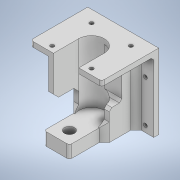
# Autodesk Inventor part: suporte barra motor 2
Saved by Autodesk Inventor 2022 (Build 260153000, 153)
## iProperties
Created: 2022-02-16
Part Number: suporte barra motor 2
Material: Genérico
Document SubType Name: Modeling
Designer: mathe
Density: 1 g/cm^3
Appearance: Padrão
Author: mathe
Autodesk Inventor part; units mm, degrees
ref_plane "YZ Plane" through (0, 0, 0) normal (1, 0, 0) x (0, 1, 0)
ref_plane "XZ Plane" through (0, 0, 0) normal (0, 1, 0) x (-1, 0, 0)
ref_plane "XY Plane" through (0, 0, 0) normal (0, 0, 1) x (1, 0, 0)
sketch "Esboço1" plane through (0, 0, 0) normal (0, 0, 1) x (1, 0, 0)
  line L0 (0, 0) -> (56, 0)
  line L1 (56, 0) -> (56, 10)
  line L2 (56, 10) -> (0, 10)
  line L3 (0, 10) -> (0, 0)
  line L4 (18, 10) -> (38, 10)
  line L5 (38, 10) -> (38, 0)
  line L6 (38, 0) -> (18, 0)
  line L7 (18, 0) -> (18, 10)
  line L8 (18, 10) -> (38, 0) construction
  line L9 (38, 10) -> (18, 0) construction
  point P0 (28, 5)
  dimension "d0" = 56
  dimension "d1" = 10
  dimension "d2" = 20
  constraints: 20 end point, 4 parallel, 2 horizontal, 2 midpoint, 2 perpendicular, 1 point on line
  measures "d0" distance of L2.end L1.end
  measures "d1" distance of L1.end L0.end
  measures "d2" distance of L5.end L6.end
extrude "Extrusão1" add sketch "Esboço1" along normal blind 4 contours L3 L2 L7 L0 | L5 L2 L1 L0
extrude "Extrusão2" add sketch "Esboço1" along normal blind 52.426 contours L7 L2 L5 L0
sketch "Esboço2" plane through (0, 10, 0) normal (0, 1, 0) x (1, 0, 0)
  line L0 (38, -52.426) -> (18, -52.426) projected
  point P0 (0, 0)
  point P1 (28, -42.426)
  point P2 (33, -52.426)
  point P3 (23, -52.426)
  dimension "d24" = 10
  measures "d24" distance from line of L0 point (28, -42.426)
hole "Furo1" at (28, 10, 42.426) direction (0, -1, 0) diameter 8 end through all
sketch "Esboço3" plane through (0, 0, 4) normal (0, 0, 1) x (1, 0, 0)
  point P0 (0, 0)
  point P1 (6.5, 5)
  point P2 (49.5, 5)
hole "Furo2" at (6.5, 5, 4) at (49.5, 5, 4) direction (0, 0, -1) diameter 3 end through all
sketch "Esboço4" plane through (0, 10, 0) normal (0, 1, 0) x (1, 0, 0)
  line L0 (56, 0) -> (0, 0) projected
  line L1 (0, 0) -> (56, 0)
  line L2 (56, 0) -> (56, -25)
  line L3 (56, -25) -> (0, -25)
  line L4 (0, -25) -> (0, 0)
  dimension "d25" = 25
  constraints: 8 end point, 2 parallel, 1 horizontal, 1 perpendicular
  measures "d25" distance of L1.end L2.end
extrude "Extrusão3" add sketch "Esboço4" along normal blind 39
sketch "Esboço5" plane through (0, 49, 0) normal (0, 1, 0) x (1, 0, 0)
  line L0 (0, -25) -> (56, -25) projected
  circle A0 centre (28, -25) radius 10
  line L1 (38, -4) -> (38, -52.426) projected
  point P0 (0, 0)
  point P1 (38, -9)
  point P2 (38, -47.426)
  point P3 (38, -25)
  point P4 (18, -25)
  constraints: 1 centre point, 1 midpoint, 1 tangent
extrude "Extrusão4" cut sketch "Esboço5" against normal blind 22 contours A0 L0 picked at (30.9515, -23.4509)
sketch "Esboço6" plane through (0, 49, 0) normal (0, 1, 0) x (1, 0, 0)
  arc A0 (38, -25) -> (18, -25) centre (28, -25) ccw projected
  line L0 (18, -25) -> (18, -52.426) projected
  line L1 (0, -25) -> (18, -25)
  line L2 (18, -25) -> (18, -45)
  line L3 (18, -45) -> (0, -45)
  line L4 (0, -45) -> (0, -25)
  line L5 (38, -25) -> (38, -52.426) projected
  line L6 (56, -25) -> (38, -25)
  line L7 (38, -25) -> (38, -45)
  line L8 (38, -45) -> (56, -45)
  line L9 (56, -45) -> (56, -25)
  circle A1 centre (43.5, -9.5) radius 1.5
  circle A2 centre (12.5, -9.5) radius 1.5
  circle A3 centre (12.5, -40.5) radius 1.5
  circle A4 centre (43.5, -40.5) radius 1.5
  point P0 (0, 0)
  point P1 (18, -47.426)
  point P2 (38, -47.426)
  dimension "d30" = 15.5
  dimension "d31" = 15.5
  dimension "d32" = 15.5
  dimension "d33" = 15.5
  dimension "d34" = 20
  dimension "d37" = 3
  dimension "d38" = 3
  dimension "d39" = 3
  dimension "d40" = 3
  dimension "d103" = 15.5
  dimension "d104" = 15.5
  constraints: 16 end point, 4 centre point, 4 coincident, 4 parallel, 3 point on line, 2 horizontal, 2 perpendicular
  measures "d30" horizontal distance of point (43.5, -9.5) A0.centre
  measures "d31" horizontal distance of A0.centre point (43.5, -9.5)
  measures "d32" horizontal distance of point (12.5, -9.5) A0.centre
  measures "d33" horizontal distance of A0.centre point (12.5, -9.5)
  measures "d34" distance of L1.end L2.end
  measures "d37" diameter of A1
  measures "d38" diameter of A2
  measures "d39" diameter of A3
  measures "d40" diameter of A4
  measures "d103" distance from line of L1 A3.centre
  measures "d104" distance from line of L6 A4.centre
extrude "Extrusão5" add sketch "Esboço6" against normal up to surface (22 mm away) contours L0 L3 L4 L1 | L6 L9 L8 L5 | A3 | A4
extrude "Extrusão6" cut sketch "Esboço6" against normal blind 20 contours A1 | A2 | A3 | A4
sketch "Esboço7" plane through (0, 0, 0) normal (-1, 0, 0) x (0, 0, 1)
  line L0 (4, 0) -> (4, 10) projected
  line L1 (45, 49) -> (45, 27) projected
  line L2 (4, 10) -> (45, 10)
  line L3 (45, 10) -> (45, 45)
  line L4 (45, 45) -> (4, 45)
  line L5 (4, 45) -> (4, 10)
  line L6 (0, 49) -> (45, 49) projected
  point P0 (0, 0)
  dimension "d43" = 4
  constraints: 8 end point, 2 parallel, 1 horizontal, 1 perpendicular, 1 point on line
  measures "d43" distance between parallel lines of L6 L4
extrude "Extrusão7" cut sketch "Esboço7" against normal blind 14
sketch "Esboço8" plane through (56, 0, 4) normal (1, 0, 0) x (0, 0, -1)
  line L0 (4, 0) -> (0, 0) projected
  line L1 (-41, 49) -> (-41, 27) projected
  line L2 (0, 0) -> (-41, 0)
  line L3 (-41, 0) -> (-41, 45)
  line L4 (-41, 45) -> (0, 45)
  line L5 (0, 45) -> (0, 0)
  line L6 (-41, 49) -> (4, 49) projected
  dimension "d46" = 4
  constraints: 8 end point, 2 parallel, 1 horizontal, 1 perpendicular, 1 point on line
  measures "d46" distance between parallel lines of L6 L4
extrude "Extrusão8" cut sketch "Esboço8" against normal blind 14
sketch "Esboço9" plane through (0, 27, 0) normal (0, 1, 0) x (1, 0, 0)
  line L0 (38, -25) -> (18, -25) projected
  circle A0 centre (28, -25) radius 10
  point P0 (0, 0)
  constraints: 1 centre point, 1 midpoint
extrude "Extrusão9" cut sketch "Esboço9" against normal up to surface (17 mm away) contours L0 A0 picked at (30.9515, -23.4509)
sketch "Esboço10" plane through (0, 10, 0) normal (0, -1, 0) x (1, 0, 0)
  line L0 (18, 25) -> (14, 25) projected
  line L1 (14, 4) -> (14, 9.5) projected
  line L2 (18, 25) -> (14, 25)
  line L3 (14, 25) -> (14, 4)
  line L4 (14, 4) -> (18, 4)
  line L5 (18, 4) -> (18, 25)
  line L6 (38, 25) -> (42, 25) projected
  line L7 (38, 4) -> (56, 4) projected
  line L8 (42, 25) -> (38, 25)
  line L9 (38, 25) -> (38, 4)
  line L10 (38, 4) -> (42, 4)
  line L11 (42, 4) -> (42, 25)
  point P0 (0, 0)
  constraints: 16 end point, 4 parallel, 2 horizontal, 2 perpendicular
extrude "Extrusão10" add sketch "Esboço10" along normal blind 10
chamfer "Chanfro2" distance 4 angle 45 8 edges at (42, 22.5, 4) (38, 5, 25) (18, 5, 25) (14, 22.5, 4) (16, 27, 25) (40, 27, 25) (40, 27, 45) (16, 27, 45)
fillet "Arredondamento1" radius 2 4 edges at (18, 5, 52.426) (38, 5, 52.426) (0, 47, 45) (56, 47, 45)
sketch "Esboço11" plane through (0, 0, 4) normal (0, 0, 1) x (1, 0, 0)
  circle A0 centre (6.5, 5) radius 1.5 projected
  line L0 (6.5, 5) -> (6.5, 38)
  point P0 (0, 0)
  point P1 (49.5, 38)
  dimension "d57" = 33
  constraints: 2 end point, 1 coincident, 1 vertical
  measures "d57" distance of L0.start L0.end
hole "Furo3" at (6.5, 38, 4) at (49.5, 38, 4) direction (0, 0, -1) diameter 3 end through all
sketch "Esboço12" plane through (0, 49, 0) normal (0, 1, 0) x (1, 0, 0)
  line L0 (0, 0) -> (56, 0)
  line L1 (56, 0) -> (56, -45)
  line L2 (56, -45) -> (0, -45)
  line L3 (0, -45) -> (0, 0)
  constraints: 8 end point, 2 parallel, 1 horizontal, 1 perpendicular
extrude "Extrusão11" add sketch "Esboço12" along normal blind 10
fillet "Arredondamento2" radius 2 2 edges at (56, 54, 45) (0, 54, 45)
sketch "Esboço13" plane through (12.5, 45, 9.5) normal (0, -1, 0) x (1, 0, 0)
  circle A0 centre (0, 0) radius 1.5 projected
  circle A1 centre (0, 0) radius 1.5
  circle A2 centre (0, 31) radius 1.5 projected
  circle A3 centre (0, 31) radius 1.5
  circle A4 centre (31, 31) radius 1.5 projected
  circle A5 centre (31, 31) radius 1.5
  circle A6 centre (31, 0) radius 1.5 projected
  circle A7 centre (31, 0) radius 1.5
  point P0 (-12.5, -9.5)
  point P1 (1.5, 0)
  point P2 (1.5, 31)
  point P3 (29.5, 0)
  constraints: 4 coincident, 4 horizontal alignment, 3 centre point, 2 other
extrude "Extrusão12" cut sketch "Esboço13" against normal through all
sketch "Esboço14" plane through (56, 0, 4) normal (1, 0, 0) x (0, 0, -1)
  line L0 (0, 0) -> (0, 45) projected
  line L1 (0, 45) -> (-45.5354, 45)
  line L2 (-45.5354, 45) -> (-45.5354, 55)
  line L3 (-45.5354, 55) -> (0, 55)
  line L4 (0, 55) -> (0, 45)
  line L5 (-39, 59) -> (4, 59) projected
  point P0 (4, 0)
  dimension "d70" = 4
  constraints: 8 end point, 2 parallel, 1 horizontal, 1 perpendicular
  measures "d70" distance between parallel lines of L5 L3
extrude "Extrusão13" cut sketch "Esboço14" against normal blind 14
sketch "Esboço15" plane through (0, 0, 0) normal (-1, 0, 0) x (0, 0, 1)
  line L0 (4, 45) -> (8, 45) projected
  line L1 (4, 45) -> (52.4988, 45)
  line L2 (52.4988, 45) -> (52.4988, 55)
  line L3 (52.4988, 55) -> (4, 55)
  line L4 (4, 55) -> (4, 45)
  line L5 (0, 59) -> (43, 59) projected
  point P0 (0, 0)
  dimension "d73" = 4
  constraints: 8 end point, 2 parallel, 1 horizontal, 1 perpendicular
  measures "d73" distance between parallel lines of L5 L3
extrude "Extrusão14" cut sketch "Esboço15" against normal blind 14
chamfer "Chanfro3" distance 4 angle 45 2 edges at (14, 50, 4) (42, 50, 4)
sketch "Esboço16" plane through (0, 49, 0) normal (0, -1, 0) x (1, 0, 0)
  arc A0 (18, 25) -> (38, 25) centre (28, 25) ccw projected
  arc A1 (18, 25) -> (38, 25) centre (28, 25) ccw
  line L0 (38, 25) -> (38, 50.426)
  line L1 (38, 25) -> (38, 45) projected
  line L2 (18, 29) -> (18, 50.426) projected
  line L3 (38, 50.426) -> (18, 50.426)
  line L4 (18, 50.426) -> (18, 29)
  line L5 (18, 45) -> (18, 25) projected
  line L6 (18, 29) -> (18, 25)
  point P0 (0, 0)
  constraints: 9 end point, 3 collinear, 2 point on circle, 1 centre point, 1 coincident, 1 perpendicular
extrude "Extrusão15" cut sketch "Esboço16" against normal through all
chamfer "Chanfro4" distance 4 angle 45 2 edges at (16.0001, 10, 25) (39.9999, 10, 25)
sketch "Esboço17" plane through (42, 0, 4) normal (1, 0, 0) x (0, 0, -1)
  line L0 (-36.5, 55) -> (-5.5, 55) projected
  line L1 (-36.5, 55) -> (-34, 55)
  line L2 (-34, 55) -> (-34, 51)
  line L3 (-34, 51) -> (-39, 51)
  line L4 (-39, 51) -> (-39, 55)
  line L5 (-41, 55) -> (-36.5, 55) projected
  line L6 (-36.5, 55) -> (-39, 55)
  line L7 (-5.5, 55) -> (-3, 55)
  line L8 (-3, 55) -> (-3, 51)
  line L9 (-3, 51) -> (-8, 51)
  line L10 (-8, 51) -> (-8, 55)
  line L11 (-5.5, 55) -> (-8, 55)
  point P0 (4, 0)
  point P1 (-5.5, 55)
  point P2 (-8, 55)
  dimension "d84" = 2.5
  dimension "d85" = 4
  dimension "d86" = 5
  dimension "d87" = 2.5
  dimension "d88" = 4
  dimension "d89" = 5
  constraints: 20 end point, 6 perpendicular, 2 point on line, 2 vertical
  measures "d84" distance of L0.start L1.end
  measures "d85" distance of L1.end L2.end
  measures "d86" distance of L2.end L3.end
  measures "d87" distance of L7.start L7.end
  measures "d88" distance of L7.end L8.end
  measures "d89" distance of L8.end L9.end
extrude "Extrusão16" cut sketch "Esboço17" along normal mid plane 2
sketch "Esboço18" plane through (14, 0, 0) normal (-1, 0, 0) x (0, 0, 1)
  line L0 (9.5, 55) -> (40.5, 55) projected
  line L1 (40.5, 55) -> (43, 55)
  line L2 (40.5, 55) -> (45, 55) projected
  line L3 (43, 55) -> (43, 51)
  line L4 (43, 51) -> (38, 51)
  line L5 (38, 51) -> (38, 55)
  line L6 (38, 55) -> (40.5, 55)
  line L7 (9.5, 55) -> (12, 55)
  line L8 (12, 55) -> (12, 51)
  line L9 (12, 51) -> (7, 51)
  line L10 (7, 51) -> (7, 55)
  line L11 (7, 55) -> (9.5, 55)
  point P0 (0, 0)
  dimension "d92" = 2.5
  dimension "d93" = 4
  dimension "d94" = 5
  dimension "d95" = 2.5
  dimension "d96" = 4
  dimension "d97" = 5
  constraints: 20 end point, 6 perpendicular, 3 point on line, 2 collinear
  measures "d92" distance of L0.end L1.end
  measures "d93" distance of L1.end L3.end
  measures "d94" distance of L3.end L4.end
  measures "d95" distance of L7.start L7.end
  measures "d96" distance of L7.end L8.end
  measures "d97" distance of L8.end L9.end
extrude "Extrusão17" cut sketch "Esboço18" along normal mid plane 2
chamfer "Chanfro5" distance 2 angle 45 2 edges at (51, 55, 4) (5, 55, 4)
sketch "Esboço19" plane through (38, 31, 45) normal (0, 0, 1) x (1, 0, 0)
  line L0 (4, 0) -> (4, 24) projected
  line L1 (4, 24) -> (-10, 24)
  line L2 (-10, 24) -> (-10, -8)
  line L3 (-10, -8) -> (4, -8)
  line L4 (4, -8) -> (4, 24)
  point P0 (-38, -31)
  dimension "d105" = 14
  constraints: 8 end point, 2 parallel, 1 horizontal, 1 perpendicular
  measures "d105" distance of L3.end L2.end
extrude "Extrusão18" cut sketch "Esboço19" against normal up to surface (30 mm away)
chamfer "Chanfro6" distance 2 angle 45 2 edges at (40, 23.0001, 25) (35, 23, 15)
